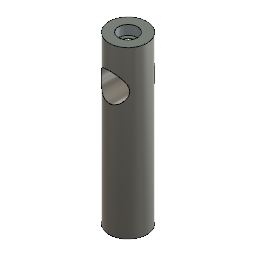
ConnectorV322mmbearinghole (Autodesk Fusion 360 archive; units mm, degrees)
design "Encoder Attachment"
Autodesk Fusion 360 part; units mm, degrees
sketch "Sketch1" plane through (0, 0, 0) normal (0, 1, 0) x (1, 0, 0)
  circle A0 centre (0, 0) radius 4
  dimension "d1" = 8
  constraint coincident A0.centre origin
  measures "d1" diameter of A0
extrude "Extrude1" add sketch "Sketch1" along normal blind 35
sketch "Sketch2" plane through (0, 0, 0) normal (0, 0, 1) x (1, 0, 0)
  circle A0 centre (0, 27) radius 3
  line L0 (4, 35) -> (-4, 35)
  dimension "d4" = 6
  dimension "d6" = 8
  measures "d4" diameter of A0
  measures "d6" distance of A0.centre L0
extrude "Extrude2" cut sketch "Sketch2" along normal through all and the other way through all
sketch "Sketch3" plane through (0, 35, 0) normal (0, 1, 0) x (-1, 0, 0)
  circle A0 centre (0, 0) radius 4
sketch "Sketch4" plane through (0, 35, 0) normal (0, 1, 0) x (-1, 0, 0)
  circle A0 centre (0, 0) radius 2
  dimension "d7" = 4
  constraint coincident A0.centre origin
  measures "d7" diameter of A0
extrude "Extrude3" cut sketch "Sketch4" against normal blind 2
hole "Hole1" at (0, 33, 0) direction (0, -1, 0) diameter 2.529 depth 5.592 tip angle 118
thread "Thread1" "ISO Metric profile 3.0 M3x0.5 6H" major diameter 3.086 minor diameter 2.529 pitch 0.5 angle 60 resizes the face on face at (-1.2645, 31.9068, 0)

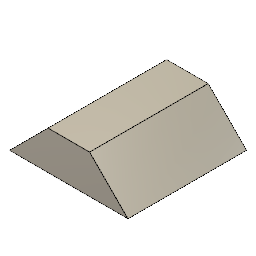
design "Triangle"
Autodesk Fusion 360 part; units mm, degrees
sketch "Sketch1" plane through (0, 0, 0) normal (0, 0, 1) x (1, 0, 0)
  line L0 (0, 0) -> (-4, 0)
  line L1 (-4, 0) -> (-1.9924, 2.0076)
  line L2 (-4, 0) -> (-1.7412, 0) construction
  line L3 (-1.9924, 2.0076) -> (0, 0)
  dimension "d1" = 4
  dimension "d2" = 45
  constraint coincident L0.start L3.end
  constraint horizontal L0
  constraint horizontal L2
  measures "d1" distance of L0.start L0.end
  measures "d2" angle of L1 L2
extrude "Extrude1" add sketch "Sketch1" along normal blind 4
sketch "Sketch2" plane through (0, 0, 4) normal (0, 0, 1) x (1, 0, 0)
  line L0 (-1.9924, 2.0076) -> (-4, 0)
  line L1 (-4, 0) -> (0, 0)
  line L2 (0, 0) -> (-1.9924, 2.0076)
  line L3 (-1.9924, 2.0076) -> (-2.7022, 1.3032)
  line L4 (-1.2933, 1.3032) -> (-1.9924, 2.0076)
  line L5 (-2.7022, 1.3032) -> (-1.2933, 1.3032)
  dimension "d5" = 1
  constraint coincident L0.start L2.end
  constraint perpendicular L2 L3
  constraint coincident L2 L4.start
  constraint parallel L2 L4
  constraint horizontal L5
  measures "d5" distance of L0.start L3.end
extrude "Extrude2" cut sketch "Sketch2" against normal blind 5 contours L0 L2 L4 L5

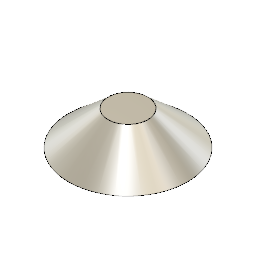
design "Flat Cone"
Autodesk Fusion 360 part; units mm, degrees
sketch "Sketch2" plane through (0, 0, 0) normal (0, 0, 1) x (1, 0, 0)
  line L0 (0, 0) -> (3, 0)
  line L1 (3, 0) -> (1, 1.7209)
  line L2 (1, 1.7209) -> (0, 1.7209)
  line L3 (0, 1.7209) -> (0, 0)
  dimension "d2" = 3
  dimension "d4" = 1
  constraint coincident L0.start L3.end
  constraint horizontal L0
  constraint horizontal L2
  constraint perpendicular L0 L3
  measures "d2" distance of L0.start L0.end
  measures "d4" distance of L1.end L2.end
revolve "Revolve1" add sketch "Sketch2" angle 360 about axis through (0, 1.7209, 0) along (0, -1, 0)
